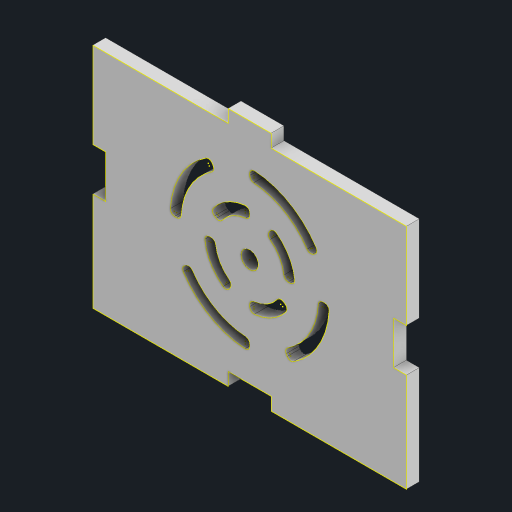
# Autodesk Inventor part: right
Saved by Autodesk Inventor 2023 (Build 270158000, 158)
## iProperties
Created: 2024-07-21
Part Number: right
Material: Generic
Document SubType Name: Modeling
Designer: Orsted
Density: 1 g/cm^3
Appearance: Default
Author: Orsted
Autodesk Inventor part; units mm, degrees
ref_plane "YZ Plane" through (0, 0, 0) normal (1, 0, 0) x (0, 1, 0)
ref_plane "XZ Plane" through (0, 0, 0) normal (0, 1, 0) x (-1, 0, 0)
ref_plane "XY Plane" through (0, 0, 0) normal (0, 0, 1) x (1, 0, 0)
sketch "Sketch1" plane through (0, 0, 0) normal (0, 0, 1) x (1, 0, 0)
  line L0 (36.5, -28) -> (-36.5, -28)
  line L1 (-36.5, -28) -> (-36.5, 28)
  line L2 (-36.5, 28) -> (36.5, 28)
  line L3 (36.5, 28) -> (36.5, -28)
  line L4 (36.5, -28) -> (-36.5, 28) construction
  line L5 (-36.5, -28) -> (36.5, 28) construction
  point P0 (0, 0)
  dimension "d0" = 73
  dimension "d1" = 56
  constraints: 12 end point, 2 midpoint, 2 parallel, 1 horizontal, 1 perpendicular
  measures "d0" distance of L1.end L2.end
  measures "d1" distance of L0.end L1.end
extrude "Extrusion1" add sketch "Sketch1" along normal blind 3
sketch "Sketch2" plane through (0, 0, 0) normal (0, 0, -1) x (-1, 0, 0)
  line L0 (36.5, -5) -> (33.5, -5)
  line L1 (33.5, -5) -> (33.5, 5)
  line L2 (33.5, 5) -> (36.5, 5)
  line L3 (36.5, 5) -> (36.5, -5)
  line L4 (36.5, -5) -> (33.5, 5) construction
  line L5 (33.5, -5) -> (36.5, 5) construction
  line L6 (36.5, 28) -> (36.5, -28) projected
  circle A0 centre (0, 0) radius 2
  circle A1 centre (0, 0) radius 8
  circle A2 centre (0, 0) radius 10.5
  circle A3 centre (0, 0) radius 16
  circle A4 centre (0, 0) radius 18.5
  line L7 (0, 0) -> (0, 10.5)
  line L8 (0, 0) -> (9.0933, 5.25)
  line L9 (0, 0) -> (0, 18.5)
  line L10 (0, 0) -> (-16.0215, 9.25)
  point P0 (35, 0)
  point P1 (36.5, 0)
  point P2 (-13.8564, 8)
  point P3 (0, 16)
  point P4 (6.9282, 4)
  point P5 (0, 8)
  dimension "d4" = 3
  dimension "d5" = 10
  dimension "d6" = 4
  dimension "d7" = 16
  dimension "d8" = 21
  dimension "d9" = 32
  dimension "d10" = 37
  dimension "d11" = 60
  dimension "d12" = 60
  constraints: 20 end point, 5 centre point, 5 coincident, 4 midpoint, 4 point on circle, 2 parallel, 2 vertical, 1 horizontal, 1 perpendicular
  measures "d4" distance of L1.end L2.end
  measures "d5" distance of L0.end L1.end
  measures "d6" diameter of A0
  measures "d7" diameter of A1
  measures "d8" diameter of A2
  measures "d9" diameter of A3
  measures "d10" diameter of A4
  measures "d11" angle of L8 L7
  measures "d12" angle of L10 L9
extrude "Extrusion3" cut sketch "Sketch2" against normal through all contours A0 L10 L8 | L8 L7 A0 | A0 L7 L10 | A1 L7 A2 L8 | L10 A4 L9 A3 picked at (-14.542, 9.8763)
fillet "Fillet1" radius 1 8 edges at (13.8564, 8, 1.5) (-6.9282, 4, 1.5) (0, 8, 1.5) (16.0215, 9.25, 1.5) (0, 10.5, 1.5) (-9.0933, 5.25, 1.5) (0, 16, 1.5) (0, 18.5, 1.5)
pattern_circular "Circular Pattern1" count 4 over 360 about axis through (0, 0, 0) along (0, 0, 1) of "Extrusion3", "Fillet1"
sketch "Sketch5" plane through (0, 0, 0) normal (0, 0, -1) x (-1, 0, 0)
  line L0 (5, 25) -> (-5, 25)
  line L1 (-5, 25) -> (-5, 28)
  line L2 (-5, 28) -> (5, 28)
  line L3 (5, 28) -> (5, 25)
  line L4 (5, 25) -> (-5, 28) construction
  line L5 (-5, 25) -> (5, 28) construction
  line L6 (36.5, 28) -> (36.5, -28) projected
  line L7 (-36.5, 28) -> (36.5, 28) projected
  line L8 (5, -28) -> (-5, -28)
  line L9 (-5, -28) -> (-5, -25)
  line L10 (-5, -25) -> (5, -25)
  line L11 (5, -25) -> (5, -28)
  line L12 (5, -28) -> (-5, -25) construction
  line L13 (-5, -28) -> (5, -25) construction
  line L14 (36.5, -28) -> (-36.5, -28) projected
  line L15 (-36.5, 5) -> (-33.5, 5)
  line L16 (-33.5, 5) -> (-33.5, -5)
  line L17 (-33.5, -5) -> (-36.5, -5)
  line L18 (-36.5, -5) -> (-36.5, 5)
  line L19 (-36.5, 5) -> (-33.5, -5) construction
  line L20 (-33.5, 5) -> (-36.5, -5) construction
  line L21 (-36.5, -28) -> (-36.5, 28) projected
  line L22 (33.5, 5) -> (36.5, 5)
  line L23 (36.5, 5) -> (36.5, -5)
  line L24 (36.5, -5) -> (33.5, -5)
  line L25 (33.5, -5) -> (33.5, 5)
  line L26 (33.5, 5) -> (36.5, -5) construction
  line L27 (36.5, 5) -> (33.5, -5) construction
  point P0 (0, 0)
  point P1 (0, 26.5)
  point P2 (0, 28)
  point P3 (0, -26.5)
  point P4 (0, -28)
  point P5 (-35, 0)
  point P6 (-36.5, 0)
  point P7 (35, 0)
  point P8 (36.5, 0)
  dimension "d31" = 10
  dimension "d32" = 3
  dimension "d33" = 36.5
  dimension "d34" = 10
  dimension "d35" = 3
  dimension "d36" = 3
  dimension "d37" = 10
  dimension "d38" = 3
  dimension "d39" = 10
  constraints: 48 end point, 16 midpoint, 8 parallel, 4 horizontal, 4 perpendicular, 1 vertical alignment
  measures "d31" distance of L1.end L2.end
  measures "d32" distance of L0.end L1.end
  measures "d33" distance from line of L6 point (0, 26.5)
  measures "d34" distance of L9.end L10.end
  measures "d35" distance of L8.end L9.end
  measures "d36" distance of L16.end L17.end
  measures "d37" distance of L15.end L16.end
  measures "d38" distance of L23.end L24.end
  measures "d39" distance of L22.end L23.end
extrude "Extrusion6" cut sketch "Sketch5" against normal through all contours L0 L1 L2 L3 | L6 L24 L25 L22 | L15 L16 L17 L18 | L8 L9 L10 L11
sketch "Sketch6" plane through (0, 0, 0) normal (0, 0, -1) x (-1, 0, 0)
  line L0 (-36.5, 28) -> (-5, 28) projected
  line L1 (5, 28) -> (36.5, 28) projected
  line L2 (5, 25) -> (-5, 25) projected
  line L3 (5, 28) -> (5, 25) projected
  line L4 (-5, 25) -> (-5, 28) projected
  line L5 (-5, 28) -> (5, 28)
  line L6 (-5, 25) -> (-36.5, 25)
  line L7 (-36.5, 5) -> (-36.5, 28) projected
  line L8 (5, 25) -> (36.5, 25)
  line L9 (36.5, 28) -> (36.5, 5) projected
  point P0 (0, 0)
  constraints: 6 end point, 2 horizontal, 2 point on line
extrude "Extrusion7" add sketch "Sketch6" against normal blind 3 contours L5 L3 L2 L4
extrude "Extrusion8" cut sketch "Sketch6" against normal through all contours L0 L4 L6 L7 | L1 L9 L8 L3
sketch "Sketch7" plane through (0, 0, 3) normal (0, 0, 1) x (1, 0, 0)
  line L0 (-5, -25) -> (-5, -28) projected
  line L1 (-5, -28) -> (-36.5, -28) projected
  line L2 (-36.5, -28) -> (-36.5, -5) projected
  line L3 (-36.5, -5) -> (-33.5, -5) projected
  line L4 (-33.5, -5) -> (-33.5, 5) projected
  line L5 (-33.5, 5) -> (-36.5, 5) projected
  line L6 (-36.5, 5) -> (-36.5, 25) projected
  line L7 (-36.5, 25) -> (-5, 25) projected
  line L8 (-5, 25) -> (-5, 28) projected
  line L9 (-5, 28) -> (5, 28) projected
  line L10 (5, 28) -> (5, 25) projected
  line L11 (5, 25) -> (36.5, 25) projected
  line L12 (36.5, 25) -> (36.5, 5) projected
  line L13 (36.5, 5) -> (33.5, 5) projected
  line L14 (33.5, 5) -> (33.5, -5) projected
  line L15 (33.5, -5) -> (36.5, -5) projected
  line L16 (36.5, -5) -> (36.5, -28) projected
  line L17 (36.5, -28) -> (5, -28) projected
  line L18 (5, -28) -> (5, -25) projected
  line L19 (5, -25) -> (-5, -25) projected
  arc A0 (16.9706, 0) -> (15.9723, -0.9412) centre (16.9706, -1) ccw projected
  arc A1 (8.8012, -13.3618) -> (15.9723, -0.9412) centre (0, 0) ccw projected
  arc A2 (8.8012, -13.3618) -> (8.4853, -14.6969) centre (9.3513, -14.1969) ccw projected
  line L20 (8.4853, -14.6969) -> (8.7357, -15.1307) projected
  arc A3 (8.7357, -15.1307) -> (10.1504, -15.4667) centre (9.6017, -14.6307) ccw projected
  arc A4 (10.1504, -15.4667) -> (18.4698, -1.0571) centre (0, 0) ccw projected
  arc A5 (18.4698, -1.0571) -> (17.4714, 0) centre (17.4714, -1) ccw projected
  line L21 (17.4714, 0) -> (16.9706, 0) projected
  arc A6 (6.178, 8.4901) -> (4.7236, 8.1815) centre (5.5896, 7.6815) ccw projected
  line L22 (4.7236, 8.1815) -> (4.4721, 7.746) projected
  arc A7 (4.4721, 7.746) -> (4.745, 6.4409) centre (5.3382, 7.246) ccw projected
  arc A8 (7.9505, 0.8889) -> (4.745, 6.4409) centre (0, 0) ccw projected
  arc A9 (7.9505, 0.8889) -> (8.9443, 0) centre (8.9443, 1) ccw projected
  line L23 (8.9443, 0) -> (9.4472, 0) projected
  arc A10 (9.4472, 0) -> (10.4417, 1.1053) centre (9.4472, 1) ccw projected
  arc A11 (10.4417, 1.1053) -> (6.178, 8.4901) centre (0, 0) ccw projected
  arc A12 (0, -16.9706) -> (-0.9412, -15.9723) centre (-1, -16.9706) ccw projected
  arc A13 (-13.3618, -8.8012) -> (-0.9412, -15.9723) centre (0, 0) ccw projected
  arc A14 (-13.3618, -8.8012) -> (-14.6969, -8.4853) centre (-14.1969, -9.3513) ccw projected
  line L24 (-14.6969, -8.4853) -> (-15.1307, -8.7357) projected
  arc A15 (-15.1307, -8.7357) -> (-15.4667, -10.1504) centre (-14.6307, -9.6017) ccw projected
  arc A16 (-15.4667, -10.1504) -> (-1.0571, -18.4698) centre (0, 0) ccw projected
  arc A17 (-1.0571, -18.4698) -> (0, -17.4714) centre (-1, -17.4714) ccw projected
  line L25 (0, -17.4714) -> (0, -16.9706) projected
  arc A18 (8.4901, -6.178) -> (8.1815, -4.7236) centre (7.6815, -5.5896) ccw projected
  line L26 (8.1815, -4.7236) -> (7.746, -4.4721) projected
  arc A19 (7.746, -4.4721) -> (6.4409, -4.745) centre (7.246, -5.3382) ccw projected
  arc A20 (0.8889, -7.9505) -> (6.4409, -4.745) centre (0, 0) ccw projected
  arc A21 (0.8889, -7.9505) -> (0, -8.9443) centre (1, -8.9443) ccw projected
  line L27 (0, -8.9443) -> (0, -9.4472) projected
  arc A22 (0, -9.4472) -> (1.1053, -10.4417) centre (1, -9.4472) ccw projected
  arc A23 (1.1053, -10.4417) -> (8.4901, -6.178) centre (0, 0) ccw projected
  arc A24 (-16.9706, 0) -> (-15.9723, 0.9412) centre (-16.9706, 1) ccw projected
  arc A25 (-8.8012, 13.3618) -> (-15.9723, 0.9412) centre (0, 0) ccw projected
  arc A26 (-8.8012, 13.3618) -> (-8.4853, 14.6969) centre (-9.3513, 14.1969) ccw projected
  line L28 (-8.4853, 14.6969) -> (-8.7357, 15.1307) projected
  arc A27 (-8.7357, 15.1307) -> (-10.1504, 15.4667) centre (-9.6017, 14.6307) ccw projected
  arc A28 (-10.1504, 15.4667) -> (-18.4698, 1.0571) centre (0, 0) ccw projected
  arc A29 (-18.4698, 1.0571) -> (-17.4714, 0) centre (-17.4714, 1) ccw projected
  line L29 (-17.4714, 0) -> (-16.9706, 0) projected
  arc A30 (-6.178, -8.4901) -> (-4.7236, -8.1815) centre (-5.5896, -7.6815) ccw projected
  line L30 (-4.7236, -8.1815) -> (-4.4721, -7.746) projected
  arc A31 (-4.4721, -7.746) -> (-4.745, -6.4409) centre (-5.3382, -7.246) ccw projected
  arc A32 (-7.9505, -0.8889) -> (-4.745, -6.4409) centre (0, 0) ccw projected
  arc A33 (-7.9505, -0.8889) -> (-8.9443, 0) centre (-8.9443, -1) ccw projected
  line L31 (-8.9443, 0) -> (-9.4472, 0) projected
  arc A34 (-9.4472, 0) -> (-10.4417, -1.1053) centre (-9.4472, -1) ccw projected
  arc A35 (-10.4417, -1.1053) -> (-6.178, -8.4901) centre (0, 0) ccw projected
  arc A36 (0, 16.9706) -> (0.9412, 15.9723) centre (1, 16.9706) ccw projected
  arc A37 (13.3618, 8.8012) -> (0.9412, 15.9723) centre (0, 0) ccw projected
  arc A38 (13.3618, 8.8012) -> (14.6969, 8.4853) centre (14.1969, 9.3513) ccw projected
  line L32 (14.6969, 8.4853) -> (15.1307, 8.7357) projected
  arc A39 (15.1307, 8.7357) -> (15.4667, 10.1504) centre (14.6307, 9.6017) ccw projected
  arc A40 (15.4667, 10.1504) -> (1.0571, 18.4698) centre (0, 0) ccw projected
  arc A41 (1.0571, 18.4698) -> (0, 17.4714) centre (1, 17.4714) ccw projected
  line L33 (0, 17.4714) -> (0, 16.9706) projected
  arc A42 (-8.4901, 6.178) -> (-8.1815, 4.7236) centre (-7.6815, 5.5896) ccw projected
  line L34 (-8.1815, 4.7236) -> (-7.746, 4.4721) projected
  arc A43 (-7.746, 4.4721) -> (-6.4409, 4.745) centre (-7.246, 5.3382) ccw projected
  arc A44 (-0.8889, 7.9505) -> (-6.4409, 4.745) centre (0, 0) ccw projected
  arc A45 (-0.8889, 7.9505) -> (0, 8.9443) centre (-1, 8.9443) ccw projected
  line L35 (0, 8.9443) -> (0, 9.4472) projected
  arc A46 (0, 9.4472) -> (-1.1053, 10.4417) centre (-1, 9.4472) ccw projected
  arc A47 (-1.1053, 10.4417) -> (-8.4901, 6.178) centre (0, 0) ccw projected
  circle A48 centre (0, 0) radius 2 projected
body "Solid1"
